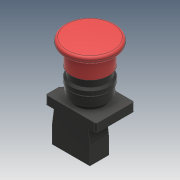
# Autodesk Inventor part: emergency-button
Saved by Autodesk Inventor 2017 (Build 210142000, 142)
## iProperties
Created: 2018-07-15
Part Number: emergency-button
Material: ABS Plastic
Document SubType Name: Modeling
Designer: Luiz Gustavo
Density: 1.06 g/cm^3
Appearance: Smooth - White
Author: Luiz Gustavo
Autodesk Inventor part; units mm, degrees
ref_plane "YZ Plane" through (0, 0, 0) normal (1, 0, 0) x (0, 1, 0)
ref_plane "XZ Plane" through (0, 0, 0) normal (0, 1, 0) x (-1, 0, 0)
ref_plane "XY Plane" through (0, 0, 0) normal (0, 0, 1) x (1, 0, 0)
sketch "Sketch1" plane through (0, 0, 0) normal (0, 0, 1) x (1, 0, 0)
  line L0 (-20.05, 15.1) -> (20.05, 15.1)
  line L1 (20.05, 15.1) -> (20.05, -15.1)
  line L2 (20.05, -15.1) -> (-20.05, -15.1)
  line L3 (-20.05, -15.1) -> (-20.05, 15.1)
  line L4 (-20.05, 15.1) -> (20.05, -15.1) construction
  line L5 (20.05, 15.1) -> (-20.05, -15.1) construction
  arc A0 (-20.05, -4.5) -> (-20.05, 4.5) centre (-22.85, 0) ccw
  line L6 (-22.85, 0) -> (-17.55, 0) construction
  line L7 (-17.55, 0) -> (0, 0) construction
  dimension "d0" = 40.1
  dimension "d1" = 30.2
  dimension "d2" = 2.5
  dimension "d3" = 9
  constraints: 16 end point, 3 horizontal, 3 point on circle, 2 midpoint, 2 parallel, 2 point on line, 1 centre point, 1 perpendicular
  measures "d0" distance of L0.start L0.end
  measures "d1" distance between parallel lines of L2 L0
  measures "d2" distance from line of L3 L6.end
  measures "d3" distance of A0.start A0.end
extrude "Extrusion1" add sketch "Sketch1" against normal blind 6.6 contours L0 L1 L2 L3 A0
sketch "Sketch2" plane through (0, 0, -6.6) normal (0, 0, -1) x (-1, 0, 0)
  line L0 (-15, -0.1) -> (15, -0.1)
  line L1 (15, -0.1) -> (15, -15.1)
  line L2 (15, -15.1) -> (-15, -15.1)
  line L3 (-15, -15.1) -> (-15, -0.1)
  line L4 (-15, -0.1) -> (15, -15.1) construction
  line L5 (15, -0.1) -> (-15, -15.1) construction
  line L6 (-20.05, -15.1) -> (20.05, -15.1) projected
  point P0 (0, 0)
  point P1 (0, -7.6)
  point P2 (0, -15.1)
  dimension "d6" = 30
  dimension "d7" = 15
  constraints: 12 end point, 4 midpoint, 2 parallel, 1 horizontal, 1 perpendicular
  measures "d6" distance of L0.start L0.end
  measures "d7" distance between parallel lines of L2 L0
extrude "Extrusion2" add sketch "Sketch2" along normal blind 25
sketch "Sketch3" plane through (0, 0, 0) normal (0, 1, 0) x (-1, 0, 0)
  line L0 (0, 0) -> (0, 43)
  line L1 (0, 0) -> (11, 0)
  line L2 (11, 0) -> (11, 4.5)
  line L3 (11, 4.5) -> (14.35, 4.5)
  line L4 (14.35, 4.5) -> (14.35, 11.1)
  line L5 (14.35, 11.1) -> (13.85, 11.1)
  line L6 (13.85, 11.1) -> (13.85, 12.1)
  line L7 (13.85, 12.1) -> (15, 12.1)
  line L8 (15, 12.1) -> (15, 15.45)
  line L9 (15, 15.45) -> (13.5, 16.95)
  line L10 (13.5, 16.95) -> (13.5, 23)
  line L11 (13.5, 23) -> (15, 23)
  line L12 (15, 23) -> (15, 37)
  line L13 (15, 37) -> (20, 37)
  line L14 (20, 37) -> (20, 42)
  line L15 (20, 43) -> (0, 43) construction
  arc A0 (20, 42) -> (0, 43) centre (0, -157.5) ccw
  line L16 (20, 42) -> (20, 43) construction
  dimension "d10" = 22
  dimension "d11" = 4.5
  dimension "d12" = 28.7
  dimension "d13" = 6.6
  dimension "d14" = 3.35
  dimension "d15" = 30
  dimension "d16" = 0.5
  dimension "d17" = 1
  dimension "d18" = 27
  dimension "d19" = 30
  dimension "d20" = 40
  dimension "d21" = 6
  dimension "d22" = 20
  dimension "d23" = 43
  dimension "d24" = 45
  dimension "d26" = 1
  constraints: 34 end point, 10 perpendicular, 4 horizontal, 2 point on circle, 2 vertical, 1 centre point, 1 parallel, 1 point on line
  measures "d10" diameter of L2 L0
  measures "d11" distance of L1.end L2.end
  measures "d12" diameter of L4 L0
  measures "d13" distance of L3.end L4.end
  measures "d14" distance of L7.end L8.end
  measures "d15" diameter of L8 L0
  measures "d16" distance of L4.end L5.end
  measures "d17" distance of L5.end L6.end
  measures "d18" diameter of L10 L0
  measures "d19" diameter of L12 L0
  measures "d20" diameter of L14 L0
  measures "d21" distance of L13.end L15.start
  measures "d22" distance between parallel lines of L15 L11
  measures "d23" distance of L0.start L0.end
  measures "d24" angle of L9 L10
  measures "d26" distance of L14.end L15.start
revolve "Revolution1" add sketch "Sketch3" angle 360 about axis through (0, 0, 0) along (0, 0, 1)
fillet "Fillet1" radius 2 3 edges at (20, 0, 42) (20, 0, 37) (15, 0, 37)
fillet "Fillet2" radius 1 4 edges at (20.05, -15.1, -3.3) (20.05, 15.1, -3.3) (-20.05, 15.1, -3.3) (-20.05, -15.1, -3.3)
sketch "Sketch4" plane through (-15, -0.1, -6.6) normal (0, 1, 0) x (1, 0, 0)
  line L0 (30, 0) -> (0, 0) projected
  line L1 (30, 0) -> (30, 25) projected
  line L2 (0, 25) -> (30, 25) projected
  line L3 (0, 0) -> (0, 25) projected
  line L4 (30, 0) -> (30, 25) projected
  line L5 (30, 11.5) -> (28.5, 0)
  line L6 (0, 11.5) -> (1.5, 0)
  line L7 (0, 25) -> (30, 25) construction
  line L8 (15, 25) -> (15, 0) construction
  point P0 (15, -6.6)
  dimension "d29" = 27
  dimension "d30" = 11.5
  constraints: 6 end point, 4 point on line, 2 midpoint, 1 other
  measures "d29" distance of L6.end L5.end
  measures "d30" vertical distance of L5.end L5.start
extrude "Extrusion3" cut sketch "Sketch4" against normal through all contours L0 L5 L1 | L0 L3 L6
body "Solid1"
